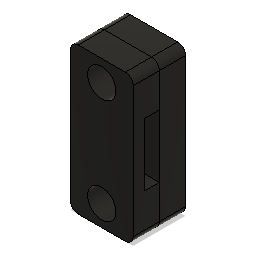
Belt_Clamp v12 (Autodesk Fusion 360 design; units mm, degrees)
Autodesk Fusion 360 part; units mm, degrees
sketch "Sketch2" plane through (0, 0, 0) normal (0, 1, 0) x (1, 0, 0)
  line L0 (0, 0) -> (2, 0)
  line L1 (2, 0) -> (2, -1.38)
  line L2 (0, 0) -> (0, -1.38)
  line L3 (-2.630986, -0.63) -> (6.308392, -0.63) construction
  circle A0 centre (2, -0.824445) radius 0.555555
  circle A1 centre (0, -0.824445) radius 0.555555
  circle A2 centre (2.4, -0.63) radius 1
  circle A3 centre (-0.4, -0.63) radius 1
  line L4 (0.676701, -0.884) -> (1.323299, -0.884)
  circle A4 centre (1.323299, -1.034) radius 0.15
  circle A5 centre (0.676701, -1.034) radius 0.15
  dimension "d10" = 2
  dimension "d11" = 0.63
  dimension "d12" = 0.75
  dimension "d13" = 1.11111
  dimension "d14" = 1.11111
  dimension "d15" = 2
  dimension "d16" = 0.4
  dimension "d17" = 0.4
  dimension "d18" = 2
  dimension "d19" = 0.254
  dimension "d20" = 0.3
  dimension "d21" = 0.3
  constraint coincident L0.start L2.start
  constraint horizontal L0
  constraint perpendicular L0 L1
  constraint perpendicular L0 L2
  constraint horizontal L3
  constraint horizontal L1.end L2.end
  constraint coincident L1.end A0
  constraint coincident L2.end A1
  constraint coincident L3 A2.centre
  constraint coincident L3 A3.centre
  constraint parallel L3 L4
  constraint tangent A2 A4
  constraint tangent L4 A5
  constraint tangent A3 A5
  constraint tangent L4 A4
  measures "d10" distance of L0.start L0.end
  measures "d11" distance of L0 L3
  measures "d12" distance of L1.end L3
  measures "d13" diameter of A0
  measures "d14" diameter of A1
  measures "d15" diameter of A2
  measures "d16" distance of L1 A2.centre
  measures "d17" distance of L2 A3.centre
  measures "d18" diameter of A3
  measures "d19" distance of L3 L4
  measures "d20" diameter of A4
  measures "d21" diameter of A5
sketch "Sketch3" plane through (0, 0, 0) normal (0, 1, 0) x (1, 0, 0)
  line L0 (0, 0) -> (6, 0)
  line L1 (6, 0) -> (6, -2.5)
  line L2 (6, -2.5) -> (0, -2.5)
  line L3 (0, -2.5) -> (0, 0)
  line L4 (0, 1) -> (6, 1)
  line L5 (6, 1) -> (6, 3.5)
  line L6 (6, 3.5) -> (0, 3.5)
  line L7 (0, 3.5) -> (0, 1)
  dimension "d30" = 2.5
  dimension "d33" = 6
  dimension "d59" = 2.5
  constraint horizontal L0
  constraint vertical L1
  constraint horizontal L2
  constraint vertical L3
  constraint coincident L0.start L3.end
  constraint horizontal L4
  constraint vertical L5
  constraint horizontal L6
  constraint vertical L7
  constraint collinear L1 L5
  constraint collinear L3 L7
  measures "d30" distance of L0.start L2.end
  measures "d33" distance of L0.start L0.end
  measures "d59" distance of L4 L6
extrude "Extrude2" add sketch "Sketch3" along normal blind 14 contours L0 L1 L2 L3 | L4 L5 L6 L7 picked at (2, -0.833333) picked at (2, 2.666667) makes body 1 at (2, 4.666667, 0) makes body 2 at (4, 4.666667, -3.5)
extrude "Extrude1" cut sketch "Sketch2" along normal blind 6 from surface at 4 contours L0 L2 A1 A3 | L0 A2 A3 L4 A4 A5 | L2 A1 | L0 L1 A0 A2 | L1 A0 picked at (0.177704, -0.097131) picked at (0.866667, -0.799333) picked at (0.12127, -0.684492) picked at (1.821685, -0.097312) picked at (1.901764, -0.981426) bodies 1
pattern_path "PathPattern2" count 10 spacing 2 from (0, 14, 0) along 1 edges at (3, 14, 0) of "Extrude1" on bodies 1
sketch "Sketch4" plane through (0, 0, 2.5) normal (0, 0, 1) x (1, 0, 0)
  line L0 (0, 0) -> (6, 0)
  line L1 (6, 0) -> (6, 14)
  line L2 (6, 14) -> (0, 14)
  line L3 (0, 14) -> (0, 0)
  circle A0 centre (3, 2) radius 1.35
  line L4 (6, 0) -> (0, 0)
  line L5 (3, 14) -> (3, 0) construction
  circle A1 centre (3, 12) radius 1.35
  dimension "d50" = 2.7
  dimension "d51" = 2
  dimension "d54" = 2.7
  dimension "d81" = 2
  constraint midpoint L2 L5.start
  constraint midpoint L4 L5.end
  constraint coincident A0.centre L5
  constraint coincident L5 A1.centre
  measures "d50" diameter of A0
  measures "d51" distance of L0 A0.centre
  measures "d54" diameter of A1
  measures "d81" distance of L2 A1.centre
extrude "Extrude5" cut sketch "Sketch4" against normal through all contours A0 | A1 picked at (2.71547, 2.724971) picked at (3.430008, 11.86736) bodies 1 2
fillet "Fillet1" radius 0.75 8 edges at (6, 14, 1.25) (0, 14, 1.25) (0, 0, 1.25) (6, 0, 1.25) (6, 14, -2.25) (0, 14, -2.25) (6, 0, -2.25) (0, 0, -2.25) on bodies 1 2
copy_body "Body->Comp1" bodies 2 removing the originals makes body 3 in component "Component"
component "Component" placed x (1, 0, 0) y (0, 1, 0) z (0, 0, 1) at (0, 0, 1)
equation "P = 2 mm"
equation "R1 = 0.3 mm"
equation "R2 = 2 mm"
equation "R3 = ( 0.555555 * 2 ) * 1 mm"
equation "b = 0.40 mm"
equation "h = 0.75 mm"
equation "i = 0.63 mm"
equation "PLD = 0.254 mm"
equation "d10 = P"
equation "d11 = i"
equation "d12 = h"
equation "d13 = R3"
equation "d14 = d13"
equation "d15 = R2"
equation "d16 = b"
equation "d17 = d16"
equation "d18 = R2"
equation "d19 = PLD"
equation "d20 = R1"
equation "d21 = d20"
equation "d54 = d50"
equation "d59 = d30"
equation "d81 = d51"
